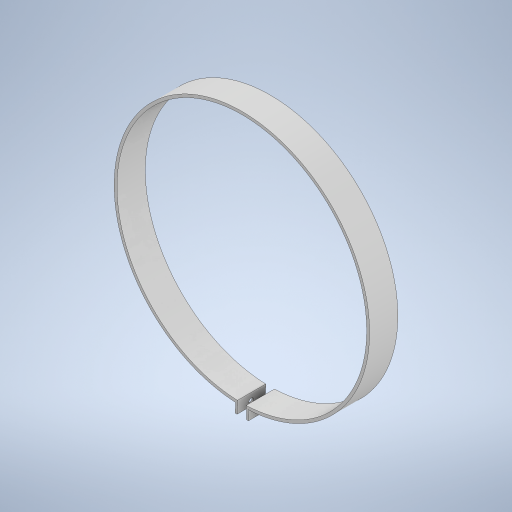
# Autodesk Inventor part: camera_robotarm
Saved by Autodesk Inventor 2024.3 (Build 283343000, 343)
## iProperties
Created: 2025-09-29
Part Number: camera_robotarm
Material: 일반
Document SubType Name: Modeling
Designer: joung
Density: 1 g/cm^3
Appearance: 기본값
Author: joung
Autodesk Inventor part; units mm, degrees
ref_plane "YZ Plane" through (0, 0, 0) normal (1, 0, 0) x (0, 1, 0)
ref_plane "XZ Plane" through (0, 0, 0) normal (0, 1, 0) x (-1, 0, 0)
ref_plane "XY Plane" through (0, 0, 0) normal (0, 0, 1) x (1, 0, 0)
sketch "스케치1" plane through (0, 0, 0) normal (0, 0, 1) x (1, 0, 0)
  arc A0 (4.6242, -132.4193) -> (-4.6242, -132.4193) centre (0, 0) ccw
  arc A1 (4.7289, -135.4175) -> (-4.7289, -135.4175) centre (0, 0) ccw
  line L0 (0, 0) -> (-4.7289, -135.4175)
  line L1 (0, 0) -> (135.5, 0) construction
  line L2 (0, 0) -> (4.7289, -135.4175)
  line L3 (0, 0) -> (135.5, 0) construction
  line L4 (-4.7289, -135.4175) -> (-5.0779, -145.4114)
  line L5 (-5.0779, -145.4114) -> (-7.0767, -145.3416)
  line L6 (-7.0767, -145.3416) -> (-6.7271, -135.3329)
  line L7 (4.7289, -135.4175) -> (5.0779, -145.4114)
  line L8 (4.7289, -135.4175) -> (14.7289, -135.4175) construction
  line L9 (5.0779, -145.4114) -> (7.0767, -145.3416)
  line L10 (7.0767, -145.3416) -> (6.7271, -135.3329)
  dimension "d0" = 265
  dimension "d1" = 3
  dimension "d2" = 92
  dimension "d3" = 88
  dimension "d4" = 10
  dimension "d5" = 2
  dimension "d6" = 90
  dimension "d7" = 90
  dimension "d8" = 10
  dimension "d9" = 88
  dimension "d10" = 2
  dimension "d11" = 90
  dimension "d12" = 90
  constraints: 22 end point, 6 point on circle, 3 equal length, 3 horizontal, 3 point on line, 2 centre point, 2 perpendicular, 1 coincident
  measures "d0" diameter of A0
  measures "d1" radial gap between concentric circles of A0 A1
  measures "d2" angle of L0 L1
  measures "d3" angle of L2 L3
  measures "d4" distance of L0.end L4.end
  measures "d5" distance of L4.end L5.end
  measures "d6" angle of L4 L5
  measures "d7" angle of L5 L6
  measures "d8" distance of L2.end L7.end
  measures "d9" angle of L7 L8
  measures "d10" distance of L7.end L9.end
  measures "d11" angle of L9 L7
  measures "d12" angle of L10 L9
extrude "돌출1" add sketch "스케치1" along normal blind 30 contours A0 L0 A1 L2 | A1 L10 L9 L7 | L4 L5 L6 A1
sketch "스케치2" plane through (6.7271, -135.3329, 30) normal (0.9994, 0.0349, 0) x (0, 0, -1)
  line L0 (30, -10.0148) -> (0, -10.0148) projected
  line L1 (15, -10.0148) -> (15, -5.0148)
  circle A0 centre (15, -5.0148) radius 2.6
  point P0 (30, 135.4852)
  dimension "d15" = 5
  dimension "d16" = 5.2
  constraints: 2 end point, 1 centre point, 1 coincident, 1 midpoint, 1 vertical
  measures "d15" distance of L1.start L1.end
  measures "d16" diameter of A0
extrude "돌출2" cut sketch "스케치2" against normal up to surface (2 mm away)
sketch "스케치3" plane through (-7.0767, -145.3416, 0) normal (-0.9994, 0.0349, 0) x (0, 0, 1)
  line L0 (0, 0) -> (30, 0) projected
  line L1 (15, 0) -> (15, 5)
  line L2 (15, 0) -> (20, 0) construction
  circle A0 centre (15, 5) radius 2.6
  point P0 (0, 145.5)
  dimension "d19" = 5
  dimension "d20" = 90
  dimension "d21" = 5.2
  constraints: 4 end point, 1 centre point, 1 coincident, 1 horizontal, 1 midpoint, 1 perpendicular, 1 vertical
  measures "d19" distance of L1.start L1.end
  measures "d20" angle of L2 L1
  measures "d21" diameter of A0
extrude "돌출3" cut sketch "스케치3" against normal up to surface (2 mm away)
